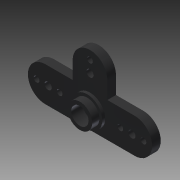
# Autodesk Inventor part: servo arm BMS-630MG tripple
Saved by Autodesk Inventor 2013 (Build 170138000, 138)
## iProperties
Created: 2014-10-08
Part Number: servo arm BMS-630MG tripple
Material: Generic
Document SubType Name: Modeling
Designer: Masta
Density: 1 g/cm^3
Author: Masta
Autodesk Inventor part; units mm, degrees
ref_plane "YZ Plane" through (0, 0, 0) normal (1, 0, 0) x (0, 1, 0)
ref_plane "XZ Plane" through (0, 0, 0) normal (0, 1, 0) x (-1, 0, 0)
ref_plane "XY Plane" through (0, 0, 0) normal (0, 0, 1) x (1, 0, 0)
sketch "Sketch1" plane through (0, 0, 0) normal (0, 1, 0) x (-1, 0, 0)
  circle A0 centre (0, 0) radius 6
  line L0 (0, 0) -> (6, 0) construction
  line L1 (0, 0) -> (0, 6) construction
  circle A1 centre (15.5, 0) radius 6
  circle A2 centre (31, 0) radius 6
  circle A3 centre (0, 12) radius 6
  circle A4 centre (15.5, 12) radius 6
  circle A5 centre (31, 12) radius 6
  circle A6 centre (15.5, 0) radius 5.25
  line L2 (0, 6) -> (31, 6)
  line L3 (0, -6) -> (31, -6)
  line L4 (9.5, 12) -> (9.5, 0)
  line L5 (21.5, 12) -> (21.5, 0)
  circle A7 centre (15.5, 0) radius 4.25
  point P0 (37, 0)
  point P1 (6, 12)
  point P2 (37, 12)
  dimension "d1" = 12
  dimension "d4" = 15.5
  dimension "d7" = 12
  dimension "d10" = 10.5
  dimension "d17" = 8.5
  constraints: 12 end point, 10 point on circle, 6 centre point, 5 tangent, 3 coincident, 2 horizontal, 2 horizontal alignment, 1 line through centre, 1 parallel, 1 perpendicular, 1 point on line, 1 vertical, 18 other
  measures "d1" diameter of A0
  measures "d4" distance of L0.start A1.centre
  measures "d7" distance of L0.start point (0, 12)
  measures "d10" diameter of A6
  measures "d17" diameter of A7
extrude "Extrusion1" add sketch "Sketch1" along normal blind 3 contours A0 | A0 L2 L4 A1 L3 | L4 A4 L2 | L2 A1 L4 | A1 | A1 L5 L2 A2 L3 | L2 L5 A1 | A4 | A4 L5 L2 | A2 | A6 | A7
extrude "Extrusion2" add sketch "Sketch1" along normal blind 3.5 and the other way blind 1 contours A6 | A7
extrude "Extrusion3" add sketch "Sketch1" against normal blind 3.5 contours A7
sketch "Sketch2" plane through (0, 3, 0) normal (0, 1, 0) x (1, 0, 0)
  circle A0 centre (-15.5, 0) radius 5.25 projected
  arc A1 (-21.5, -12) -> (-9.5, -12) centre (-15.5, -12) ccw projected
  arc A2 (0, -6) -> (0, 6) centre (0, 0) ccw projected
  arc A3 (-31, 6) -> (-31, -6) centre (-31, 0) ccw projected
  line L0 (-37, 0) -> (6, 0) construction
  line L1 (-15.5, 0) -> (-15.5, -18) construction
  point P0 (-26, 0)
  point P1 (-30, 0)
  point P2 (-34, 0)
  point P3 (-15.5, -15)
  point P4 (-15.5, -11)
  point P5 (-5, 0)
  point P6 (-1, 0)
  point P7 (3, 0)
  dimension "d20" = 11
  dimension "d22" = 15
  dimension "d23" = 10.5
  dimension "d24" = 14.5
  dimension "d25" = 18.5
  constraints: 5 point on line, 4 end point, 3 point on circle, 3 symmetric about line
  measures "d20" distance from line of point (-15.5, -11) L0
  measures "d22" distance from line of point (-15.5, -15) L0
  measures "d23" distance from line of point (-26, 0) L1
  measures "d24" distance from line of L1 point (-30, 0)
  measures "d25" distance from line of L1 point (-34, 0)
hole "Hole1" at (-26, 3, 0) at (-34, 3, 0) at (-15.5, 3, 15) at (3, 3, 0) at (-5, 3, 0) direction (0, -1, 0) diameter 2 end through all
hole "Hole2" at (-30, 3, 0) at (-15.5, 3, 11) at (-1, 3, 0) direction (0, -1, 0) diameter 2.5 end through all
hole "Hole3" at (-15.5, 3.5, 0) direction (0, -1, 0) diameter 5.5 depth 1
hole "Hole4" at (-15.5, 3.5, 0) direction (0, -1, 0) diameter 3 end through all
hole "Hole5" at (-15.5, -3.5, 0) direction (0, 1, 0) diameter 6 depth 4
body "Solid1"
